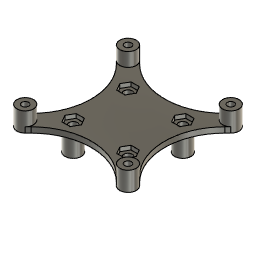
pix32 stands v4 (Autodesk Fusion 360 design; units mm, degrees)
Autodesk Fusion 360 part; units mm, degrees
note: some values were not read from the file. Set by a fixed rule: which sketch regions a step uses.
sketch "Sketch1" plane through (0, 0, 0) normal (0, 0, 1) x (1, 0, 0)
  circle A0 centre (0, 0) radius 1.25
  circle A1 centre (37.5, 0) radius 1.25
  line L0 (0, 0) -> (37.5, 0) construction
  line L1 (18.75, 0) -> (18.75, 21) construction
  line L2 (0, 18.75) -> (42, 18.75) construction
  circle A2 centre (8.75, 8.75) radius 1.5
  circle A3 centre (28.75, 8.75) radius 1.5
  line L3 (6.6287, 10.8713) -> (-2.1213, 2.1213)
  arc A4 (-2.1213, 2.1213) -> (2.1213, -2.1213) centre (0, 0) ccw
  line L4 (2.1213, -2.1213) -> (10.8713, 6.6287)
  arc A5 (10.8713, 6.6287) -> (6.6287, 10.8713) centre (8.75, 8.75) ccw
  line L5 (8.75, 8.75) -> (0, 0) construction
  line L6 (8.75, 5.75) -> (28.75, 5.75)
  arc A6 (28.75, 5.75) -> (28.75, 11.75) centre (28.75, 8.75) ccw
  line L7 (28.75, 11.75) -> (8.75, 11.75)
  arc A7 (8.75, 11.75) -> (8.75, 5.75) centre (8.75, 8.75) ccw
  line L8 (8.75, 8.75) -> (28.75, 8.75) construction
  line L9 (39.6213, 2.1213) -> (30.8713, 10.8713)
  arc A8 (30.8713, 10.8713) -> (26.6287, 6.6287) centre (28.75, 8.75) ccw
  line L10 (26.6287, 6.6287) -> (35.3787, -2.1213)
  arc A9 (35.3787, -2.1213) -> (39.6213, 2.1213) centre (37.5, 0) ccw
  line L11 (37.5, 0) -> (28.75, 8.75) construction
  line L12 (11.75, 8.75) -> (10.25, 11.3481)
  line L13 (10.25, 11.3481) -> (7.25, 11.3481)
  line L14 (7.25, 11.3481) -> (5.75, 8.75)
  line L15 (5.75, 8.75) -> (7.25, 6.1519)
  line L16 (7.25, 6.1519) -> (10.25, 6.1519)
  line L17 (10.25, 6.1519) -> (11.75, 8.75)
  line L18 (25.75, 8.75) -> (27.25, 6.1519)
  line L19 (27.25, 6.1519) -> (30.25, 6.1519)
  line L20 (30.25, 6.1519) -> (31.75, 8.75)
  line L21 (31.75, 8.75) -> (30.25, 11.3481)
  line L22 (30.25, 11.3481) -> (27.25, 11.3481)
  line L23 (27.25, 11.3481) -> (25.75, 8.75)
  circle A10 centre (0, 0) radius 3
  circle A11 centre (37.5, 0) radius 3
  arc A12 (2.1213, 39.6213) -> (-2.1213, 35.3787) centre (0, 37.5) ccw
  arc A13 (28.75, 25.75) -> (28.75, 31.75) centre (28.75, 28.75) ccw
  arc A14 (26.6287, 30.8713) -> (30.8713, 26.6287) centre (28.75, 28.75) ccw
  circle A15 centre (37.5, 37.5) radius 1.25
  line L24 (30.25, 26.1519) -> (27.25, 26.1519)
  line L25 (28.75, 25.75) -> (8.75, 25.75)
  line L26 (27.25, 31.3481) -> (30.25, 31.3481)
  circle A16 centre (8.75, 28.75) radius 1.5
  line L27 (27.25, 26.1519) -> (25.75, 28.75)
  circle A17 centre (28.75, 28.75) radius 1.5
  line L28 (5.75, 28.75) -> (7.25, 31.3481)
  circle A18 centre (0, 37.5) radius 1.25
  line L29 (30.25, 31.3481) -> (31.75, 28.75)
  line L30 (10.25, 31.3481) -> (11.75, 28.75)
  line L31 (8.75, 28.75) -> (0, 37.5) construction
  circle A19 centre (0, 37.5) radius 3
  line L32 (39.6213, 35.3787) -> (30.8713, 26.6287)
  line L33 (10.25, 26.1519) -> (7.25, 26.1519)
  line L34 (7.25, 26.1519) -> (5.75, 28.75)
  line L35 (11.75, 28.75) -> (10.25, 26.1519)
  line L36 (6.6287, 26.6287) -> (-2.1213, 35.3787)
  arc A20 (8.75, 31.75) -> (8.75, 25.75) centre (8.75, 28.75) ccw
  line L37 (8.75, 28.75) -> (28.75, 28.75) construction
  arc A21 (39.6213, 35.3787) -> (35.3787, 39.6213) centre (37.5, 37.5) ccw
  circle A22 centre (37.5, 37.5) radius 3
  line L38 (7.25, 31.3481) -> (10.25, 31.3481)
  arc A23 (6.6287, 26.6287) -> (10.8713, 30.8713) centre (8.75, 28.75) ccw
  line L39 (26.6287, 30.8713) -> (35.3787, 39.6213)
  line L40 (0, 37.5) -> (37.5, 37.5) construction
  line L41 (25.75, 28.75) -> (27.25, 31.3481)
  line L42 (2.1213, 39.6213) -> (10.8713, 30.8713)
  line L43 (31.75, 28.75) -> (30.25, 26.1519)
  line L44 (8.75, 31.75) -> (28.75, 31.75)
  line L45 (37.5, 37.5) -> (28.75, 28.75) construction
  line L46 (5.75, 28.75) -> (5.75, 8.75)
  arc A24 (5.75, 8.75) -> (11.75, 8.75) centre (8.75, 8.75) ccw
  line L47 (11.75, 8.75) -> (11.75, 28.75)
  arc A25 (11.75, 28.75) -> (5.75, 28.75) centre (8.75, 28.75) ccw
  line L48 (8.75, 28.75) -> (8.75, 8.75) construction
  line L49 (25.75, 28.75) -> (25.75, 8.75)
  arc A26 (25.75, 8.75) -> (31.75, 8.75) centre (28.75, 8.75) ccw
  line L50 (31.75, 8.75) -> (31.75, 28.75)
  arc A27 (31.75, 28.75) -> (25.75, 28.75) centre (28.75, 28.75) ccw
  line L51 (28.75, 28.75) -> (28.75, 8.75) construction
  point P0 (8.75, 8.75)
  point P1 (28.75, 8.75)
  point P2 (8.75, 28.75)
  point P3 (28.75, 28.75)
  point P4 (18.75, 37.5)
  point P5 (0, 37.5)
  dimension "d7" = 2.5
  dimension "d8" = 2.5
  dimension "d9" = 37.5
  dimension "d10" = 18.75
  dimension "d11" = 3
  dimension "d12" = 3
  dimension "d13" = 10
  dimension "d14" = 10
  dimension "d15" = 10
  dimension "d16" = 10
  dimension "d17" = 6
  dimension "d18" = 6
  dimension "d19" = 6
  dimension "d20" = 6
  dimension "d21" = 6
  constraint coincident A0.centre L0.start
  constraint coincident A1.centre L0.end
  constraint horizontal L0
  constraint midpoint L0 L1.start
  constraint perpendicular L0 L1
  constraint perpendicular L1 L2
  constraint tangent L3 A4
  constraint tangent A4 L4
  constraint parallel L3 L4
  constraint tangent L4 A5
  constraint tangent L3 A5
  constraint coincident P0 A2.centre
  constraint tangent L6 A6
  constraint tangent A6 L7
  constraint parallel L6 L7
  constraint tangent L7 A7
  constraint tangent L6 A7
  constraint coincident P1 A3.centre
  constraint horizontal L8
  constraint tangent L9 A8
  constraint tangent A8 L10
  constraint parallel L9 L10
  constraint tangent L10 A9
  constraint tangent L9 A9
  constraint coincident A5 L12.start
  constraint coincident L8 L12.start
  constraint coincident A8 L18.start
  constraint coincident L8 L18.start
  constraint concentric A9 A11
  constraint symmetric A0.centre L2 P5
  constraint symmetric A0 L2 A18
  constraint symmetric A1 L2 A15
  constraint symmetric A1.centre L2 A15.centre
  constraint symmetric L1.start L2 P4
  constraint symmetric L2 A2 A16
  constraint symmetric L2 A3 A17
  constraint symmetric L2 L3.start L36.start
  constraint symmetric L2 L3.end A12.end
  constraint symmetric L2 A4.end A12.start
  constraint symmetric L2 L4.end A23.end
  constraint symmetric L2 A4 A12
  constraint symmetric L2 A5 A23
  constraint symmetric L2 L6.start A20.start
  constraint symmetric L2 L6.end A13.end
  constraint symmetric L2 A6.end A13.start
  constraint symmetric L2 L7.end L25.end
  constraint symmetric L2 A6 A13
  constraint symmetric L2 A7 A20
  constraint symmetric L2 L9.start L32.start
  constraint symmetric L2 L9.end A14.end
  constraint symmetric L2 A8.end A14.start
  constraint symmetric L2 L10.end A21.end
  constraint symmetric L2 A8 A14
  constraint symmetric L2 A9 A21
  constraint symmetric L2 L12.start L30.end
  constraint symmetric L2 L12.end L33.start
  constraint symmetric L2 L13.end L33.end
  constraint symmetric L2 L14.end L28.start
  constraint symmetric L2 L15.end L28.end
  constraint symmetric L2 L16.end L30.start
  constraint symmetric L2 P0 P2
  constraint symmetric L2 L18.start L27.end
  constraint symmetric L2 L18.end L26.start
  constraint symmetric L2 L19.end L26.end
  constraint symmetric L2 L20.end L29.end
  constraint symmetric L2 L21.end L24.start
  constraint symmetric L2 L22.end L24.end
  constraint symmetric L2 P1 P3
  constraint symmetric L2 A10 A19
  constraint symmetric L2 A11 A22
  constraint tangent L46 A24
  constraint tangent A24 L47
  constraint parallel L46 L47
  constraint tangent L47 A25
  constraint tangent L46 A25
  constraint perpendicular L8 L48
  constraint coincident P2 A16.centre
  constraint tangent L49 A26
  constraint tangent A26 L50
  constraint parallel L49 L50
  constraint tangent L50 A27
  constraint tangent L49 A27
  constraint perpendicular L8 L51
  constraint coincident P3 A13.centre
  measures "d7" diameter of A0
  measures "d8" diameter of A1
  measures "d9" distance of A0.centre A1.centre
  measures "d10" distance of L0 L2
  measures "d11" diameter of A2
  measures "d12" diameter of A3
  measures "d13" distance of L2 P0
  measures "d14" distance of L1 P0
  measures "d15" distance of L1 P1
  measures "d16" distance of L2 P1
  measures "d17" diameter of A4
  measures "d18" diameter of A6
  measures "d19" diameter of A8
  measures "d20" diameter of A24
  measures "d21" diameter of A26
extrude "Extrude1" add sketch "Sketch1" along normal blind 2
extrude "Extrude2" add sketch "Sketch1" along normal blind 7 contours A4 A10 | A12 A19 | A9 A11 | A21 A22
extrude "Extrude3" add sketch "Sketch1" against normal blind 8 contours A5 A7 L14 | A5 A7 L13 | L12 L13 L14 L15 L16 L17 | A7 L15 A24 | A5 L12 | A7 L16 A24 | L34 A20 A23 | L28 A20 A25 | L28 L30 L33 L34 L35 L38 | A5 L17 A24 | L33 A20 A23 | A20 L38 A25 | L35 A23 | L30 A23 A25 | A6 A8 L22 | A8 L18 A26 | L18 L19 L20 L21 L22 L23 | A8 L23 | A6 L19 A26 | A6 A8 L21 | A13 A14 L24 | A14 L27 | L24 L26 L27 L29 L41 L43 | A14 L41 A27 | A6 L20 A26 | A13 L26 A27 | A13 A14 L43 | A13 L29 A27
extrude "Extrude4" cut sketch "Sketch1" along normal blind 1.5 from surface at 0.5 contours L12 L13 L14 L15 L16 L17 | L28 L30 L33 L34 L35 L38 | L18 L19 L20 L21 L22 L23 | L24 L26 L27 L29 L41 L43
fillet "Fillet1" radius 22 8 edges at (5.75, 27.5074, 1) (5.75, 9.9926, 1) (9.9926, 31.75, 1) (27.5074, 31.75, 1) (31.75, 27.5074, 1) (31.75, 9.9926, 1) (9.9926, 5.75, 1) (27.5074, 5.75, 1)
sketch "Sketch2" plane through (0, 0, 0) normal (0, 0, 1) x (1, 0, 0)
equation "d10 = ( 37.5 / 2 ) * 1 mm"
